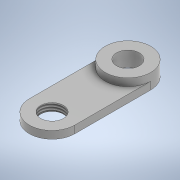
# Autodesk Inventor part: linkToActuator5
Saved by Autodesk Inventor 2021 (Build 250183000, 183)
## iProperties
Created: 2021-01-03
Part Number: linkToActuator5
Material: Generic
Document SubType Name: Modeling
Designer: awitc
Density: 1 g/cm^3
Appearance: Smooth - Medium Gray
Author: awitc
Autodesk Inventor part; units mm, degrees
ref_plane "YZ Plane" through (0, 0, 0) normal (1, 0, 0) x (0, 1, 0)
ref_plane "XZ Plane" through (0, 0, 0) normal (0, 1, 0) x (-1, 0, 0)
ref_plane "XY Plane" through (0, 0, 0) normal (0, 0, 1) x (1, 0, 0)
sketch "Sketch2" plane through (0, 0, 0) normal (0, 1, 0) x (-1, 0, 0)
  circle A0 centre (3, 0) radius 1.5
  circle A1 centre (3, 0) radius 3
  circle A2 centre (3, -10) radius 1.5
  circle A3 centre (3, -10) radius 3
  line L0 (6, 0) -> (6, -10)
  line L1 (0, -10) -> (0, 0)
  dimension "d40" = 6
  dimension "d39" = 3
  dimension "d41" = 3
  dimension "d42" = 6
  constraints: 4 end point, 3 centre point, 2 coincident, 2 point on circle, 2 tangent, 1 parallel, 1 vertical, 3 other
  measures "d39" diameter of A0
  measures "d41" diameter of A2
  measures "d42" diameter of A3
extrude "Extrusion6" add sketch "Sketch2" along normal blind 1 contours A1 | L0 A3 L1 A1
extrude "Extrusion7" add sketch "Sketch2" along normal blind 2 contours A3
thread "Thread1" size "M3x0.35" class "6H" standard "ANSI Metric M Profile" length 1
body "Solid5"
